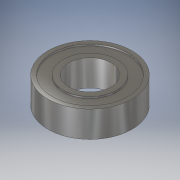
# Autodesk Inventor part: Ball Bearing 8 x 16 x 5
Saved by Autodesk Inventor 2019 (Build 230136000, 136)
## iProperties
Created: 2020-11-22
Part Number: Ball Bearing 8 x 16 x 5
Material: Stainless Steel
Document SubType Name: Modeling
Designer: asus
Density: 8 g/cm^3
Appearance: Chrome - Polished
Author: asus
Autodesk Inventor part; units mm, degrees
ref_plane "YZ Plane" through (0, 0, 0) normal (1, 0, 0) x (0, 1, 0)
ref_plane "XZ Plane" through (0, 0, 0) normal (0, 1, 0) x (-1, 0, 0)
ref_plane "XY Plane" through (0, 0, 0) normal (0, 0, 1) x (1, 0, 0)
sketch "Sketch1" plane through (0, 0, 0) normal (1, 0, 0) x (0, 1, 0)
  line L0 (-5, -4.25) -> (-5, -5.9)
  line L1 (0, -4) -> (0, -5.1)
  line L2 (0, -5.1) -> (-0.3, -5.1)
  line L3 (-0.3, -5.1) -> (-0.3, -7.2)
  line L4 (-0.3, -7.2) -> (0, -7.2)
  line L5 (0, -7.2) -> (0, -8)
  line L6 (0, -8) -> (-5, -8)
  line L7 (-5, -8) -> (-5, -7.2)
  line L8 (-5, -7.2) -> (-4.7, -7.2)
  line L9 (-4.7, -7.2) -> (-4.7, -5.1)
  line L10 (-4.7, -5.1) -> (-5, -5.1)
  line L11 (-5, -5.1) -> (-5, -4)
  line L12 (-5, -4) -> (0, -4)
  line L13 (0, 0) -> (-5.2831, 0)
  constraints: 28 end point, 1 horizontal
revolve "Revolution1" add sketch "Sketch1" angle 360 about axis through (0, 0, 0) along (0, -1, 0)
body "Solid1"
